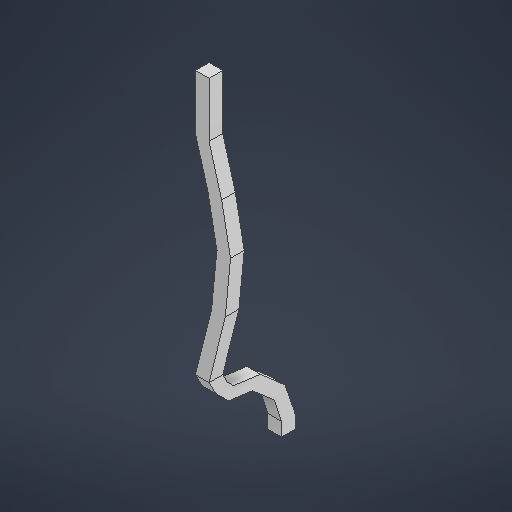
# Autodesk Inventor part: jst-vh-2p_wire
Saved by Autodesk Inventor 2025.2 (Build 292293000, 293)
## iProperties
Created: 2025-12-13
Part Number: jst-vh-2p_wire
Material: Generic
Document SubType Name: Modeling
Designer: sam
Density: 1 g/cm^3
Appearance: Default
Author: sam
Autodesk Inventor part; units mm, degrees
ref_plane "YZ Plane" through (0, 0, 0) normal (1, 0, 0) x (0, 1, 0)
ref_plane "XZ Plane" through (0, 0, 0) normal (0, 1, 0) x (-1, 0, 0)
ref_plane "XY Plane" through (0, 0, 0) normal (0, 0, 1) x (1, 0, 0)
sketch "Sketch1" plane through (0, 0, 0) normal (0, 0, 1) x (1, 0, 0)
  line L0 (0, 0) -> (1, 0)
  line L1 (0.5, 0) -> (0.5, 15.3)
  line L2 (0.5, 0) -> (15.8, 0) construction
  line L3 (0, 15.3) -> (1, 15.3)
  line L4 (1, 0) -> (2.1839, 4.7541)
  line L5 (2.1839, 4.7541) -> (2.5706, 8.6743)
  line L6 (1, 15.3) -> (1.9212, 12.0419)
  line L7 (1.9212, 12.0419) -> (2.5706, 8.6743)
  line L8 (0, 15.3) -> (0.9212, 12.0419)
  line L9 (0.9212, 12.0419) -> (1.5706, 8.6743)
  line L10 (1.1839, 4.7541) -> (1.5706, 8.6743)
  line L11 (0, 0) -> (1.1839, 4.7541)
  point P0 (0.5, 0)
  point P1 (0.5, 15.3)
  dimension "d0" = 1
  dimension "d1" = 15.3
  dimension "d2" = 90
  dimension "d4" = 0
  dimension "d5" = 1
  dimension "d6" = 0.5
  constraints: 24 end point, 3 horizontal, 1 midpoint, 1 perpendicular, 1 vertical
  measures "d0" distance of L0.start L0.end
  measures "d1" distance of L1.start L1.end
  measures "d2" angle of L2 L1
  measures "d4" distance of L1.start point (0.5, 0)
  measures "d5" distance of L3.start L3.end
  measures "d6" distance of L1.end L3.end
extrude "Extrusion1" add sketch "Sketch1" along normal blind 1 contours L11 L1 L0 | L1 L11 L10 L9 L8 L3 L6 L7 L5 L4 L0 | L8 L3 L1
sketch "Sketch2" plane through (-0.71, 15.3, 0) normal (0, 1, 0) x (1, 0, 0)
  line L0 (1.71, 0) -> (0.71, 0) projected
  line L1 (1.71, -1) -> (0.71, -1) projected
  line L2 (1.71, 0) -> (1.71, -1) projected
  line L3 (0.71, 0) -> (0.71, -1) projected
extrude "Extrusion2" add sketch "Sketch2" along normal blind 4
sketch "Sketch4" plane through (1, 15.3, 0) normal (1, 0, 0) x (0, 0, -1)
  line L0 (-1, 4) -> (0, 4) projected
  line L1 (-1, -15.3) -> (0, -15.3)
  line L2 (4.3, -20.4) -> (3.7812, -18.7843)
  line L3 (3.7812, -18.7843) -> (2.1719, -17.398)
  line L4 (2.1719, -17.398) -> (0.4286, -17.1646)
  line L5 (0.4286, -17.1646) -> (-0.5, -16.2449)
  line L6 (-0.5, -16.2449) -> (-1, -15.3)
  line L7 (5.3, -20.4) -> (4.5609, -18.2271)
  line L8 (4.5609, -18.2271) -> (2.7638, -16.6488)
  line L9 (2.7638, -16.6488) -> (0.7923, -16.3849)
  line L10 (0.7923, -16.3849) -> (0.3338, -15.9308)
  line L11 (0.3338, -15.9308) -> (0, -15.3)
  line L12 (4.3, -20.4) -> (5.3, -20.4)
  line L13 (0, -15.3) -> (-1, -15.3) projected
  point P0 (0, 3)
  point P1 (0, -15.3)
  dimension "d13" = 1
  dimension "d22" = 5.1
  dimension "d23" = 5.1
  dimension "d24" = 5.3
  dimension "d25" = 5.3
  dimension "d28" = 0
  dimension "d29" = 0
  constraints: 24 end point, 1 horizontal
  measures "d13" distance of L1.start L1.end
  measures "d22" vertical distance of L2.start L1.start
  measures "d23" vertical distance of L7.start L1.end
  measures "d24" horizontal distance of L2.start L1.start
  measures "d25" horizontal distance of L1.end L7.start
  measures "d28" distance from line of L13 L1.start
  measures "d29" distance of L13.start L1.end
extrude "Extrusion4" add sketch "Sketch4" against normal blind 1
sketch "Sketch6" plane through (1, -5.1, -5.3) normal (0, -1, 0) x (1, 0, 0)
  line L0 (0, 1) -> (0, 0) projected
  line L1 (0, 1) -> (-1, 1) projected
  line L2 (-1, 0) -> (-1, 1) projected
  line L3 (0, 0) -> (-1, 0) projected
  point P0 (-1, 5.3)
extrude "Extrusion6" add sketch "Sketch6" along normal blind 1
equation "\"d23\" = d22"
equation "\"d25\" = d24"
body "Solid1"
